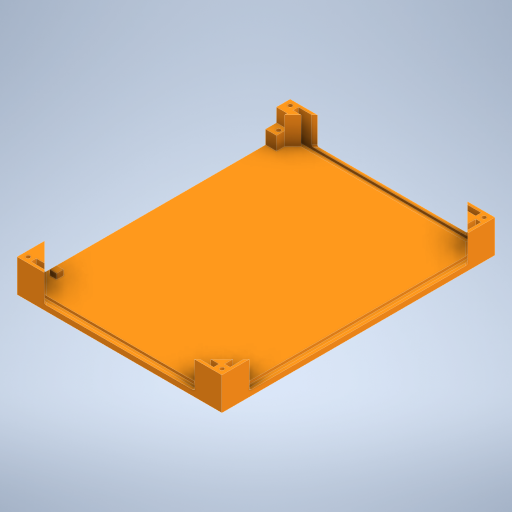
# Autodesk Inventor part: Cabinet
Saved by Autodesk Inventor 2024.3 (Build 283343000, 343)
## iProperties
Created: 2025-03-25
Part Number: Cabinet
Material: Všeobecné
Document SubType Name: Modeling
Designer: admin
Density: 1 g/cm^3
Appearance: Oranžová
Author: admin
Autodesk Inventor part; units mm, degrees
ref_plane "YZ Plane" through (0, 0, 0) normal (1, 0, 0) x (0, 1, 0)
sketch "Náčrt1" plane through (0, 0, 0) normal (0, 1, 0) x (-1, 0, 0)
  line L0 (75, 100) -> (-75, 100)
  line L1 (-75, 100) -> (-75, -100)
  line L2 (-75, -100) -> (75, -100)
  line L3 (75, -100) -> (75, 100)
  line L4 (105, 0) -> (-105, 0) projected
  line L5 (0, -140) -> (0, 140) projected
  point P0 (0, 0)
  dimension "d0" = 200
  dimension "d1" = 150
  constraints: 8 end point, 2 parallel, 1 horizontal, 1 perpendicular, 2 other
  measures "d0" distance of L2.end L0.start
  measures "d1" distance of L0.start L0.end
extrude "Vysunutí1" add sketch "Náčrt1" along normal blind 4
sketch "Náčrt2" plane through (0, 4, 0) normal (0, 1, 0) x (1, 0, 0)
  line L0 (-75, -100) -> (-75, -80)
  line L1 (-75, -100) -> (-55, -100)
  line L2 (-75, 100) -> (-75, -100) projected
  line L3 (-75, -100) -> (75, -100) projected
  line L4 (-67, -98) -> (-57, -98)
  line L5 (-61, -94) -> (-67, -94)
  line L6 (-67, -94) -> (-67, -98)
  line L7 (-55, -100) -> (-57, -98)
  line L8 (-61, -94) -> (-75, -80)
  line L9 (55, -100) -> (75, -100)
  line L10 (75, -100) -> (75, -80)
  line L11 (75, -100) -> (75, 100) projected
  line L12 (57, -98) -> (67, -98)
  line L13 (67, -98) -> (67, -94)
  line L14 (67, -94) -> (61, -94)
  line L15 (57, -98) -> (55, -100)
  line L16 (69, -92) -> (73, -92)
  line L17 (73, -92) -> (73, -82)
  line L18 (69, -86) -> (69, -92)
  line L19 (75, -80) -> (73, -82)
  line L20 (69, -86) -> (61, -94)
  point P0 (0, 0)
  point P1 (55, -100)
  dimension "d4" = 20
  dimension "d17" = 4
  dimension "d18" = 2
  dimension "d19" = 8
  dimension "d20" = 10
  dimension "d21" = 6
  dimension "d66" = 20
  dimension "d67" = 20
  dimension "d70" = 2
  dimension "d71" = 10
  dimension "d72" = 8
  dimension "d74" = 4
  dimension "d75" = 6
  dimension "d77" = 10
  dimension "d78" = 2
  dimension "d79" = 8
  dimension "d80" = 4
  dimension "d81" = 6
  constraints: 36 end point, 5 horizontal, 4 collinear, 4 perpendicular, 3 parallel, 1 point on line, 1 vertical
  measures "d4" distance of L0.end L0.start
  measures "d17" distance of L5.end L4.start
  measures "d18" distance between parallel lines of L1 L4
  measures "d19" distance between parallel lines of L0 L6
  measures "d20" distance of L4.start L4.end
  measures "d21" distance of L5.start L5.end
  measures "d66" distance of L9.start L9.end
  measures "d67" distance of L9.end L10.end
  measures "d70" distance between parallel lines of L3 L12
  measures "d71" distance of L12.start L12.end
  measures "d72" distance between parallel lines of L10 L13
  measures "d74" distance of L12.end L13.end
  measures "d75" distance of L13.end L14.end
  measures "d77" distance of L17.end L16.end
  measures "d78" distance between parallel lines of L11 L17
  measures "d79" distance between parallel lines of L9 L16
  measures "d80" distance of L16.start L16.end
  measures "d81" distance of L18.start L16.start
extrude "Vysunutí7" add sketch "Náčrt2" along normal blind 20
mirror "Zrcadlit5" about plane through (0, 0, 0) normal (0, 0, 1) of "Vysunutí7"
ref_plane "Pracovní rovina2" through (0, 14, 0) normal (0, 1, 0) x (1, 0, 0)
sketch "Náčrt11" plane through (0, 0, 0) normal (0, -1, 0) x (1, 0, 0)
  line L0 (75, -100) -> (-75, -100) projected
  line L1 (-75, -100) -> (-75, 100) projected
  point P0 (0, 0)
  point P1 (-71, -96)
  dimension "d100" = 4
  dimension "d101" = 4
  measures "d100" distance from line of L0 point (-71, -96)
  measures "d101" distance from line of L1 point (-71, -96)
hole "Díra4" at (-71, 0, -96) direction (0, 1, 0) diameter 3 end through all countersink diameter 6.3 countersink angle 90 clearance for "Šroub se zápustnou hlavou ISO 2009/7046" size "M3" standard "ISO"
pattern_circular "Kruhové pole1" count 2 over 360 about axis through (0, -10, 0) along (0, 1, 0) of "Díra4"
mirror "Zrcadlit6" about plane through (0, 0, 0) normal (0, 0, 1) of "Kruhové pole1", "Díra4"
sketch "Náčrt12" plane through (0, 4, 0) normal (0, 1, 0) x (1, 0, 0)
  line L0 (-67, -98) -> (67, -98)
  line L1 (67, -98) -> (67, -94)
  line L2 (67, -94) -> (-67, -94)
  line L3 (-67, -94) -> (-67, -98)
  line L4 (-67, -98) -> (-67, -94) projected
  line L5 (67, -94) -> (67, -98) projected
  line L6 (61, -94) -> (67, -94) projected
  line L7 (67, -98) -> (57, -98) projected
  point P0 (0, 0)
  constraints: 8 end point, 4 collinear, 2 parallel, 1 horizontal, 1 perpendicular
extrude "Vysunutí9" cut sketch "Náčrt12" against normal blind 2
mirror "Zrcadlit7" about plane through (0, 0, 0) normal (0, 0, 1) of "Vysunutí9"
sketch "Náčrt13" plane through (0, 4, 0) normal (0, 1, 0) x (1, 0, 0)
  line L0 (69, -92) -> (73, -92)
  line L1 (73, -92) -> (73, 92)
  line L2 (73, 92) -> (69, 92)
  line L3 (69, 92) -> (69, -92)
  line L4 (73, -92) -> (69, -92) projected
  line L5 (73, 92) -> (69, 92) projected
  line L6 (73, 82) -> (73, 92) projected
  line L7 (69, 92) -> (69, 86) projected
  point P0 (0, 0)
  constraints: 8 end point, 4 collinear, 2 parallel, 1 horizontal, 1 perpendicular
extrude "Vysunutí10" cut sketch "Náčrt13" against normal blind 2
sketch "Náčrt14" plane through (0, 4, 0) normal (0, 1, 0) x (1, 0, 0)
  line L0 (-71, -80) -> (-66, -80)
  line L1 (-66, -80) -> (-66, -75)
  line L2 (-66, -75) -> (-71, -75)
  line L3 (-71, -75) -> (-71, -80)
  line L4 (-75, 80) -> (-75, -80) projected
  line L5 (-75, -100) -> (-55, -100) projected
  point P0 (0, 0)
  dimension "d116" = 5
  dimension "d117" = 5
  dimension "d118" = 4
  dimension "d119" = 20
  constraints: 8 end point, 2 parallel, 1 horizontal, 1 perpendicular
  measures "d116" distance of L0.end L1.end
  measures "d117" distance of L1.end L2.end
  measures "d118" distance between parallel lines of L4 L3
  measures "d119" distance between parallel lines of L5 L0
extrude "Vysunutí11" add sketch "Náčrt14" along normal blind 4
fillet "Zaoblení1" radius 1 9 edges at (-56, 4, -99) (56, 4, -99) (65, 4, -90) (74, 4, -81) (-56, 4, 99) (-68, 4, 87) (65, 4, 90) (74, 4, 81) (56, 4, 99)
sketch "Náčrt15" plane through (-75, 24, -100) normal (0, 1, 0) x (1, 0, 0)
  line L0 (0, -10) -> (8, -10)
  line L1 (8, -10) -> (8, -20)
  line L2 (8, -20) -> (0, -20)
  line L3 (0, -20) -> (0, -10)
  line L4 (0, -20) -> (0, 0) projected
  point P0 (75, -100)
  dimension "d123" = 8
  dimension "d124" = 10
  constraints: 8 end point, 2 parallel, 1 collinear, 1 horizontal, 1 perpendicular
  measures "d123" distance of L1.end L2.end
  measures "d124" distance of L0.end L1.end
extrude "Vysunutí12" cut sketch "Náčrt15" against normal up to surface (20 mm away)
sketch "Náčrt16" plane through (0, 4, 0) normal (0, 1, 0) x (1, 0, 0)
  line L0 (-75, 90) -> (-75, -78.5858) projected
  line L1 (-75, 90) -> (-67, 90)
  line L2 (-67, 90) -> (-67, 82)
  line L3 (-67, 82) -> (-75, 82)
  line L4 (-75, 82) -> (-75, 90)
  line L5 (-75, 90) -> (-67, 90) projected
  line L6 (-67, 90) -> (-67, 88) projected
  point P0 (0, 0)
  dimension "d142" = 8
  constraints: 8 end point, 3 collinear, 2 parallel, 1 horizontal, 1 perpendicular
  measures "d142" distance of L1.end L2.end
ref_plane "Pracovní rovina3" through (0, 14, 0) normal (0, 1, 0) x (1, 0, 0)
extrude "Vysunutí14" add sketch "Náčrt16" along normal blind 10
sketch "Náčrt18" plane through (0, 14, 0) normal (0, 1, 0) x (1, 0, 0)
  line L0 (-67, 82) -> (-67, 88) projected
  line L1 (-75, 82) -> (-67, 82) projected
  point P0 (0, 0)
  point P1 (-69.5, 86)
  dimension "d145" = 2.5
  dimension "d146" = 4
  measures "d145" distance from line of L0 point (-69.5, 86)
  measures "d146" distance from line of L1 point (-69.5, 86)
hole "Díra6" at (-69.5, 14, -86) direction (0, -1, 0) diameter 3 depth 5
